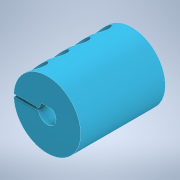
# Autodesk Inventor part: NEMA17toACMETr8
Saved by Autodesk Inventor 2021 (Build 250183000, 183)
## iProperties
Created: 2021-03-11
Part Number: NEMA17toACMETr8
Material: Generic
Document SubType Name: Modeling
Designer: elmar
Density: 1 g/cm^3
Appearance: Turquoise
Author: elmar
Autodesk Inventor part; units mm, degrees
ref_plane "YZ Plane" through (0, 0, 0) normal (1, 0, 0) x (0, 1, 0)
ref_plane "XY Plane" through (0, 0, 0) normal (0, 0, 1) x (1, 0, 0)
sketch "Sketch1" plane through (0, 0, 0) normal (0, 0, 1) x (1, 0, 0)
  circle A0 centre (0, 0) radius 9.5
  line L0 (-7.5495, 5.7667) -> (-3.9295, 5.7667)
  line L1 (-3.9295, 5.7667) -> (-3.9295, 3.9067)
  line L2 (-3.9295, 3.9067) -> (-7.5495, 3.9067)
  line L3 (-7.5495, 3.9067) -> (-7.5495, 5.7667)
  line L4 (-6.8395, 3.9067) -> (-4.6395, 3.9067)
  line L5 (-4.6395, 3.9067) -> (-4.6395, -6.5933)
  line L6 (-4.6395, -6.5933) -> (-6.8395, -6.5933)
  line L7 (-6.8395, -6.5933) -> (-6.8395, 3.9067)
  line L8 (-7.7395, -3.9091) -> (-3.7395, -3.9091)
  line L9 (-3.7395, -3.9091) -> (-3.7395, -5.5091)
  line L10 (-3.7395, -5.5091) -> (-7.7395, -5.5091)
  line L11 (-7.7395, -5.5091) -> (-7.7395, -3.9091)
  line L12 (-5.7395, 3.9067) -> (-5.7395, -3.9091)
  dimension "d0" = 19
  dimension "d41" = 3.62
  dimension "d42" = 1.86
  dimension "d44" = 2.2
  dimension "d45" = 10.5
  dimension "HoleDepth" = 5.5933
  dimension "HoleOffset" = 5.7395
  dimension "d49" = 4
  dimension "d50" = 1.6
  dimension "NutDepth" = 5.5909
  dimension "d67" = 9.4158
  constraints: 26 end point, 6 parallel, 4 perpendicular, 3 horizontal, 3 midpoint, 3 point on circle, 1 centre point, 1 coincident, 1 point on line
  measures "d0" diameter of A0
  measures "d41" distance of L0.start L0.end
  measures "d42" distance of L2.end L0.start
  measures "d44" distance of L5.end L6.end
  measures "d45" distance of L6.end L4.start
  measures "HoleDepth" distance edge to line of A0 L2
  measures "HoleOffset" horizontal distance of point (0, 0) L12.start
  measures "d49" distance of L9.end L10.end
  measures "d50" distance of L10.end L8.start
  measures "NutDepth" distance edge to line of A0 L8
  measures "d67" distance between parallel lines of L2 L10
extrude "Extrusion1" add sketch "Sketch1" along normal mid plane 24
sketch "Sketch2" plane through (0, 0, 12) normal (0, 0, 1) x (1, 0, 0)
  circle A0 centre (0, 0) radius 2.5
  line L0 (-1.5, 2) -> (1.5, 2)
  dimension "d3" = 5
  dimension "d4" = 4.5
  constraints: 2 end point, 2 point on circle, 1 centre point, 1 coincident, 1 horizontal
  measures "d3" diameter of A0
extrude "Extrusion2" cut sketch "Sketch2" against normal blind 12 contours A0 L0 picked at (0.1119, 0.5076)
sketch "Sketch4" plane through (0, 0, -12) normal (0, 0, -1) x (-1, 0, 0)
  point P0 (0, 0)
hole "Hole1" at (0, 0, -12) direction (0, 0, 1) diameter 8 depth 12
sketch "Sketch5" plane through (0, 0, 0) normal (0, 1, 0) x (-1, 0, 0)
  line L0 (0, -16.3608) -> (0, 2.7268) projected
  line L1 (4, -12.366) -> (3, -12.634)
  line L2 (3, -12.634) -> (3, -13.366)
  line L3 (3, -13.366) -> (4, -13.634)
  line L4 (4, -13.634) -> (4, -12.366)
  line L5 (-9.5, -12) -> (9.5, -12) projected
  point P0 (0, 0)
  point P1 (3.5, -12.5)
  point P2 (3.5, -13.5)
  dimension "d17" = 1
  dimension "d18" = 1
  dimension "d19" = 30
  dimension "d37" = 4
  dimension "d38" = 0.5
  constraints: 8 end point, 2 midpoint, 2 point on line, 1 equal length, 1 vertical
  measures "d17" distance between parallel lines of L2 L4
  measures "d18" distance of point (3.5, -13.5) point (3.5, -12.5)
  measures "d19" angle of L3 L1
  measures "d37" distance between parallel lines of L0 L4
  measures "d38" distance from line of L5 point (3.5, -12.5)
coil "Coil1" sketch "Sketch5" operation add axis through (0, 0, -10) along (0, 0, 1) pitch 2 turns 7 hand right separate body
ref_plane "Work Plane3" through (0, 0, -12) normal (0, 0, -1) x (-1, 0, 0)
split "Split1" plane through (0, 0, -12) removes the side toward (0, 0, -1) bodies 2
split "Split2" plane through (0, 0, 0) removes the side toward (0, 0, 1) bodies 2
ref_plane "Work Plane1" through (0, 9.5, 0) normal (0, -1, 0) x (1, 0, 0)
combine bodies "Combine1" operation type add bodies to combine 1 2
sketch "Sketch3" plane through (0, 9.5, 0) normal (0, -1, 0) x (1, 0, 0)
  line L0 (9.5, 12) -> (-9.5, 12) projected
  line L1 (-9.5, -12) -> (9.5, -12) projected
  line L2 (-5.7395, 12) -> (-5.7395, -12)
  point P0 (0, 0)
  point P1 (-5.7395, 9)
  point P2 (-5.7395, 3)
  point P3 (-5.7395, -9)
  point P4 (-5.7395, -3)
  dimension "d7" = 3
  dimension "d9" = 6
  dimension "d35" = 3
  dimension "d36" = 6
  dimension "d40" = 5.7395
  constraints: 6 point on line, 2 end point, 1 vertical
  measures "d7" distance from line of L0 point (-5.739, 9)
  measures "d9" distance of point (-5.739, 3) point (-5.739, 9)
  measures "d35" distance from line of L1 point (-5.739, -9)
  measures "d36" distance of point (-5.739, -9) point (-5.739, -3)
  measures "d40" distance from line of L2 point (0, 0)
hole "Hole2" at (-5.7395, 9.5, 9) at (-5.7395, 9.5, 3) at (-5.7395, 9.5, -3) at (-5.7395, 9.5, -9) direction (0, -1, 0) diameter 2.2 end through all counterbore diameter 4.4 counterbore depth 5.5933 bodies 1 clearance for "Socket Head Cap Screw" size "M2" standard "Ansi Metric M Profile"
ref_plane "Work Plane4" through (0, -9.5, 0) normal (0, 1, 0) x (-1, 0, 0)
sketch "Sketch6" plane through (0, -9.5, 0) normal (0, 1, 0) x (-1, 0, 0)
  circle A0 centre (5.7395, -9) radius 2.2 projected
  line L0 (7.7395, -10.1547) -> (5.7395, -11.3094)
  line L1 (5.7395, -11.3094) -> (3.7395, -10.1547)
  line L2 (3.7395, -10.1547) -> (3.7395, -7.8453)
  line L3 (3.7395, -7.8453) -> (5.7395, -6.6906)
  line L4 (5.7395, -6.6906) -> (7.7395, -7.8453)
  line L5 (7.7395, -7.8453) -> (7.7395, -10.1547)
  circle A1 centre (5.7395, -3) radius 1.1 projected
  line L6 (7.7395, -1.8453) -> (7.7395, -4.1547)
  line L7 (7.7395, -4.1547) -> (5.7395, -5.3094)
  line L8 (5.7395, -5.3094) -> (3.7395, -4.1547)
  line L9 (3.7395, -4.1547) -> (3.7395, -1.8453)
  line L10 (3.7395, -1.8453) -> (5.7395, -0.6906)
  line L11 (5.7395, -0.6906) -> (7.7395, -1.8453)
  circle A2 centre (5.7395, 3) radius 1.1 projected
  line L12 (7.7395, 4.1547) -> (7.7395, 1.8453)
  line L13 (7.7395, 1.8453) -> (5.7395, 0.6906)
  line L14 (5.7395, 0.6906) -> (3.7395, 1.8453)
  line L15 (3.7395, 1.8453) -> (3.7395, 4.1547)
  line L16 (3.7395, 4.1547) -> (5.7395, 5.3094)
  line L17 (5.7395, 5.3094) -> (7.7395, 4.1547)
  circle A3 centre (5.7395, 9) radius 1.1 projected
  line L18 (7.7395, 10.1547) -> (7.7395, 7.8453)
  line L19 (7.7395, 7.8453) -> (5.7395, 6.6906)
  line L20 (5.7395, 6.6906) -> (3.7395, 7.8453)
  line L21 (3.7395, 7.8453) -> (3.7395, 10.1547)
  line L22 (3.7395, 10.1547) -> (5.7395, 11.3094)
  line L23 (5.7395, 11.3094) -> (7.7395, 10.1547)
  point P0 (0, 0)
  dimension "d48" = 4
  constraints: 48 end point, 4 coincident, 4 vertical, 3 equal length, 3 horizontal alignment, 56 other
  measures "d48" distance between parallel lines of L2 L5
extrude "Extrusion3" cut sketch "Sketch6" along normal blind 5.5909 contours L5 A0 L0 L1 L2 L3 L4 | A0 L4 L5 | L5 L0 A0 | A0 L3 L4 | L0 L1 A0 | A0 L2 L3 | L1 L2 A0 | A1 | L6 L7 L8 L9 L10 L11 | A2 | L12 L13 L14 L15 L16 L17 | A3 | L18 L19 L20 L21 L22 L23 bodies 1
sketch "Sketch7" plane through (0, 0, 0) normal (0, 0, 1) x (1, 0, 0)
  line L0 (0, 0.4) -> (-9.5, 0.4)
  line L1 (-9.5, 0.4) -> (-9.5, -0.4)
  line L2 (-9.5, -0.4) -> (0, -0.4)
  line L3 (0, -0.4) -> (0, 0.4)
  circle A0 centre (0, 0) radius 9.5 projected
  dimension "d55" = 0.8
  constraints: 8 end point, 2 parallel, 1 coincident, 1 horizontal, 1 midpoint, 1 perpendicular, 1 tangent
  measures "d55" distance of L0.end L1.end
extrude "Extrusion4" cut sketch "Sketch7" along normal through all both and the other way through all contours L3 L2 A0 L0 | A0 L1 L0 | A0 L2 L1 picked at (-3.1667, 0) bodies 1
sketch "Sketch8" plane through (0, 0, 0) normal (0, 1, 0) x (-1, 0, 0)
  line L0 (0, 0.2) -> (9.4916, 0.2)
  line L1 (9.4916, 0.2) -> (9.4916, -0.2)
  line L2 (9.4916, -0.2) -> (0, -0.2)
  line L3 (0, -0.2) -> (0, 0.2)
  line L4 (9.4916, -12) -> (9.4916, 12) projected
  point P0 (0, 0)
  point P1 (0, 0)
  dimension "d58" = 0.4
  constraints: 8 end point, 2 parallel, 1 coincident, 1 collinear, 1 horizontal, 1 midpoint, 1 perpendicular
  measures "d58" distance of L0.end L1.end
extrude "Extrusion5" cut sketch "Sketch8" against normal through all bodies 1
sketch "Sketch9" plane through (0, 0, 0) normal (0, 0, 1) x (1, 0, 0)
  arc A0 (-9.4916, -0.4) -> (0, -9.5) centre (0, 0) ccw projected
  line L0 (0, -3) -> (0, -9.5) projected
  arc A1 (-0.6178, -2.9357) -> (0, -3) centre (0, 0) ccw projected
  spline S0 degree 6 poles (-3.4681, -1.993) (-3.3547, -2.101) (-3.2362, -2.2032) (-3.1129, -2.2993) (-2.9851, -2.389) (-2.8532, -2.4719) (-2.5893, -2.6191) (-2.4576, -2.6844) (-2.3229, -2.7428) (-2.1858, -2.7942) (-2.0465, -2.8382) (-1.6939, -2.9296) (-1.4786, -2.9675) (-1.2613, -2.9875) (-1.0439, -2.9891) (-0.8287, -2.9718) (-0.6178, -2.9357) knots 0 0 0 0 0 0 0 0.296516 0.296516 0.296516 0.296516 0.296516 0.577531 0.577531 0.577531 0.577531 0.577531 1 1 1 1 1 1 1 projected
  arc A2 (-3.9799, -0.4) -> (-3.4681, -1.993) centre (0, 0) ccw projected
  line L1 (-9.4916, -0.4) -> (-3.9799, -0.4) projected
  arc A3 (-9.0648, -0.8) -> (0, -9.1) centre (0, 0) ccw
  line L2 (-9.0648, -0.8) -> (-4.3267, -0.8)
  arc A4 (-4.3267, -0.8) -> (-3.8149, -2.1923) centre (0, 0) ccw
  arc A5 (-3.8149, -2.1923) -> (0, -3.4) centre (-1.0223, 0) ccw
  line L3 (0, 0) -> (-3.8149, -2.1923)
  line L4 (-13.5844, 0) -> (2.2641, 0) projected
  dimension "d61" = 0.4
  dimension "d62" = 0.4
  dimension "d63" = 0.4
  dimension "d64" = 0.4
  constraints: 6 point on circle, 4 end point, 4 point on line, 3 centre point, 2 concentric, 1 horizontal, 1 other
  measures "d61" radial gap between concentric circles of A0 A3
  measures "d62" distance between parallel lines of L2 L1
  measures "d63" radial gap between concentric circles of A2 A4
  measures "d64" distance of L0.start A5.end
extrude "Extrusion6" add sketch "Sketch9" along normal mid plane 0.4 separate body contours L1 A2 L3 A4 L2 A3 L0 A0 | S0 A1 L0 A5 L3
equation "\"d40\" = HoleOffset"
equation "\"d31\" = HoleDepth"
equation "\"d53\" = NutDepth"
body "Solid1"
